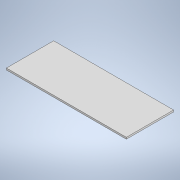
# Autodesk Inventor part: Internal hinge side verticle
Saved by Autodesk Inventor 2021 (Build 250183000, 183)
## iProperties
Created: 2020-07-02
Part Number: Internal hinge side verticle
Material: Generic
Document SubType Name: Modeling
Designer: jgray
Density: 1 g/cm^3
Appearance: Default
Author: jgray
Autodesk Inventor part; units mm, degrees
ref_plane "YZ Plane" through (0, 0, 0) normal (1, 0, 0) x (0, 1, 0)
ref_plane "XZ Plane" through (0, 0, 0) normal (0, 1, 0) x (-1, 0, 0)
ref_plane "XY Plane" through (0, 0, 0) normal (0, 0, 1) x (1, 0, 0)
sketch "Sketch1" plane through (0, 0, 0) normal (0, 1, 0) x (-1, 0, 0)
  line L0 (-174, -68.5) -> (174, -68.5)
  line L1 (174, -68.5) -> (174, 68.5)
  line L2 (174, 68.5) -> (-174, 68.5)
  line L3 (-174, 68.5) -> (-174, -68.5)
  line L4 (-174, -68.5) -> (174, 68.5) construction
  line L5 (174, -68.5) -> (-174, 68.5) construction
  point P0 (0, 0)
  dimension "d0" = 348
  dimension "d1" = 137
  constraints: 12 end point, 2 midpoint, 2 parallel, 1 horizontal, 1 perpendicular
  measures "d0" distance of L2.end L1.end
  measures "d1" distance of L1.end L0.end
extrude "Extrusion1" add sketch "Sketch1" along normal blind 5
body "Solid1"
